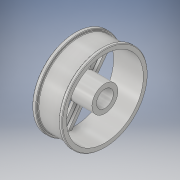
# Autodesk Inventor part: T9 Rim
Saved by Autodesk Inventor 2018 (Build 220112000, 112)
## iProperties
Created: 2018-02-18
Part Number: T9 Rim
Material: Phenolic Resin
Document SubType Name: Modeling
Designer: Blue Mist
Density: 1.38 g/cm^3
Appearance: Smooth - Light Orange
Author: Blue Mist
Autodesk Inventor part; units mm, degrees
ref_plane "YZ Plane" through (0, 0, 0) normal (1, 0, 0) x (0, 1, 0)
ref_plane "XZ Plane" through (0, 0, 0) normal (0, 1, 0) x (-1, 0, 0)
ref_plane "XY Plane" through (0, 0, 0) normal (0, 0, 1) x (1, 0, 0)
sketch "Sketch1" plane through (0, 0, 0) normal (0, 0, 1) x (1, 0, 0)
  line L0 (0, 0) -> (0, 17.653) construction
  line L1 (0, 17.907) -> (0, 21.209)
  line L2 (0.254, 21.463) -> (1.524, 21.463)
  line L3 (1.778, 21.209) -> (1.778, 18.923)
  line L4 (2.032, 18.669) -> (12.192, 18.669)
  line L5 (12.446, 18.923) -> (12.446, 21.209)
  line L6 (12.7, 21.463) -> (13.97, 21.463)
  line L7 (14.224, 21.209) -> (14.224, 17.907)
  line L8 (13.97, 17.653) -> (0.254, 17.653)
  arc A0 (13.97, 17.653) -> (14.224, 17.907) centre (13.97, 17.907) ccw
  arc A1 (14.224, 21.209) -> (13.97, 21.463) centre (13.97, 21.209) ccw
  arc A2 (12.7, 21.463) -> (12.446, 21.209) centre (12.7, 21.209) ccw
  arc A3 (12.192, 18.669) -> (12.446, 18.923) centre (12.192, 18.923) ccw
  arc A4 (1.778, 18.923) -> (2.032, 18.669) centre (2.032, 18.923) ccw
  arc A5 (1.778, 21.209) -> (1.524, 21.463) centre (1.524, 21.209) ccw
  arc A6 (0.254, 21.463) -> (0, 21.209) centre (0.254, 21.209) ccw
  arc A7 (0, 17.907) -> (0.254, 17.653) centre (0.254, 17.907) ccw
  line L9 (-2.9184, 0) -> (17.1424, 0) projected
  point P0 (0, 21.463)
  point P1 (1.778, 21.463)
  point P2 (1.778, 18.669)
  point P3 (12.446, 18.669)
  point P4 (12.446, 21.463)
  point P5 (14.224, 21.463)
  point P6 (14.224, 17.653)
  dimension "d0" = 17.653
  dimension "d1" = 3.81
  dimension "d2" = 1.778
  dimension "d3" = 2.794
  dimension "d4" = 10.668
  dimension "d5" = 2.794
  dimension "d6" = 1.778
  dimension "d7" = 3.81
  dimension "d8" = 0.254
  constraints: 19 point on line, 18 end point, 16 point on circle, 16 tangent, 8 centre point, 7 equal radius, 3 perpendicular, 1 parallel, 1 vertical
  measures "d0" distance of L0.start L0.end
  measures "d1" distance of L0.end point (0, 21.463)
  measures "d2" distance of point (0, 21.463) point (1.778, 21.463)
  measures "d3" distance of point (1.778, 21.463) point (1.778, 18.669)
  measures "d4" distance of point (1.778, 18.669) point (12.446, 18.669)
  measures "d5" distance of point (12.446, 18.669) point (12.446, 21.463)
  measures "d6" distance of point (12.446, 21.463) point (14.224, 21.463)
  measures "d7" distance of point (14.224, 21.463) point (14.224, 17.653)
  measures "d8" radius of A0
revolve "Revolution1" add sketch "Sketch1" angle 360 about axis through (-10, 0, 0) along (1, 0, 0)
sketch "Sketch2" plane through (0, 0, 0) normal (0, 0, 1) x (1, 0, 0)
  line L0 (0.254, -17.653) -> (0.254, 17.653) projected
  line L1 (0, -17.907) -> (0, 17.907) projected
  line L2 (0, -21.209) -> (0, 21.209) projected
  line L3 (13.97, -17.653) -> (13.97, 17.653) projected
  line L4 (0.254, -17.653) -> (0.254, 17.653) projected
  line L5 (13.97, 17.653) -> (0.254, 17.653) projected
  arc A0 (0.254, 21.463) -> (0, 21.209) centre (0.254, 21.209) ccw projected
  line L6 (0.254, 21.463) -> (1.524, 21.463) projected
  line L7 (0, -21.209) -> (0, 21.209) projected
  line L8 (0.254, -21.463) -> (0.254, 21.463) projected
  line L9 (1.524, -21.463) -> (1.524, 21.463) projected
  line L10 (1.778, -21.209) -> (1.778, 21.209) projected
  line L11 (14.224, -17.907) -> (14.224, 17.907) projected
  line L12 (1.524, -21.463) -> (1.524, 21.463) projected
  line L13 (14.224, -21.209) -> (14.224, 21.209) projected
  line L14 (0, 17.8534) -> (2.54, 5.969)
  line L15 (2.54, 5.969) -> (2.54, 3.8735)
  line L16 (2.54, 3.8735) -> (14.224, 3.8735)
  line L17 (14.224, 3.8735) -> (14.224, 5.969)
  line L18 (0, 17.8534) -> (1.27, 17.8534) construction
  line L19 (2.54, 5.969) -> (3.81, 5.969) construction
  line L20 (1.27, 17.653) -> (3.81, 5.969)
  line L21 (14.224, 5.969) -> (3.81, 5.969)
  line L22 (0, 17.8534) -> (1.27, 17.653)
  line L23 (-2.9079, 0) -> (17.0793, 0) projected
  point P0 (0, 0)
  dimension "d10" = 2.54
  dimension "d11" = 13.7795
  dimension "d12" = 2.54
  dimension "d13" = 11.684
  dimension "d14" = 1.27
  constraints: 18 end point, 4 point on line, 2 collinear, 2 perpendicular, 1 parallel
  measures "d10" distance from line of L1 L15.end
  measures "d11" distance from line of L5 L15.end
  measures "d12" distance from line of L1 L14.end
  measures "d13" distance from line of L5 L14.end
  measures "d14" distance of L14.end L19.end
revolve "Revolution2" add sketch "Sketch2" angle 360 about axis through (-10, 0, 0) along (1, 0, 0) contours L14 L22 L8 L0 | L0 L5 L20 L9 L14 | L8 L22 L5 | L9 L20 L10 L14 | L10 L20 L21 L3 L16 L15 L14 | L3 L21 L11 L16
sketch "Sketch3" plane through (0, 0, 0) normal (-1, 0, 0) x (0, 0, 1)
  circle A0 centre (0, 0) radius 17.8534 construction
  circle A1 centre (0, 0) radius 5.969 construction
  line L0 (5.969, 1.016) -> (5.8819, 1.016)
  circle A2 centre (0, 0) radius 5.969 projected
  line L1 (5.969, -1.016) -> (5.8819, -1.016)
  line L2 (5.969, -1.016) -> (17.6237, -1.016)
  circle A3 centre (0, 0) radius 17.653 projected
  line L3 (5.969, 1.016) -> (17.6237, 1.016)
  arc A4 (17.6237, -1.016) -> (17.6237, 1.016) centre (0, 0) ccw
  arc A5 (5.8819, -1.016) -> (5.8819, 1.016) centre (0, 0) ccw
  dimension "d16" = 1.016
  dimension "d17" = 1.016
  constraints: 8 end point, 8 point on circle, 2 centre point, 2 concentric, 2 horizontal, 2 parallel
  measures "d16" vertical distance of point (0, 0) L0.start
  measures "d17" vertical distance of point (0, 0) L1.start
extrude "Extrusion1" cut sketch "Sketch3" against normal blind 25.4 contours L3 A3 L2 L1 A2 L0 picked at (9.8507, 0.7907)
pattern_circular "Circular Pattern1" count 5 over 360 about axis through (-10, 0, 0) along (1, 0, 0) of "Extrusion1"
sketch "Sketch4" plane through (0, 0, 0) normal (-1, 0, 0) x (0, 0, 1)
  line L0 (-5.3557, 2.6353) -> (-14.8551, 9.537) projected
  line L1 (-14.8551, -9.537) -> (-5.3557, -2.6353) projected
  arc A0 (-14.8551, 9.537) -> (-14.8551, -9.537) centre (0, 0) ccw projected
  arc A1 (-5.3557, 2.6353) -> (-5.3557, -2.6353) centre (0, 0) ccw projected
  line L2 (-14.4076, 7.0142) -> (-7.1395, 1.7336)
  line L3 (-7.1395, 1.7336) -> (-5.9096, 0.84)
  arc A2 (-5.3557, 2.6353) -> (-5.3557, -2.6353) centre (0, 0) ccw projected
  line L4 (-14.4076, 7.0142) -> (-15.7438, 7.985)
  line L5 (-14.0745, -6.7722) -> (-7.4288, -1.9438)
  line L6 (-7.4288, -1.9438) -> (-5.9096, -0.84)
  line L7 (-14.0745, -6.7722) -> (-15.7438, -7.985)
  arc A3 (-5.9096, 0.84) -> (-5.9096, -0.84) centre (0, 0) ccw
  arc A4 (-15.7438, 7.985) -> (-15.7438, -7.985) centre (0, 0) ccw
  dimension "d23" = 1.778
  dimension "d24" = 1.778
  dimension "d25" = 1.778
  dimension "d26" = 1.778
  constraints: 12 end point, 7 point on circle, 3 point on line, 2 centre point
  measures "d23" distance from line of L0 L2.end
  measures "d24" distance from line of L0 L2.start
  measures "d25" distance from line of L1 L5.end
  measures "d26" distance from line of L1 L5.start
extrude "Extrusion2" cut sketch "Sketch4" against normal blind 25.4 contours A1 L6 L5 L7 A0 L4 L2 L3
pattern_circular "Circular Pattern2" count 5 over 360 about axis through (-10, 0, 0) along (1, 0, 0) of "Extrusion2"
sketch "Sketch5" plane through (14.224, 0, 0) normal (1, 0, 0) x (0, 0, -1)
  circle A0 centre (0, 0) radius 21.463 projected
extrude "Extrusion3" cut sketch "Sketch5" against normal blind 0.508
sketch "Sketch6" plane through (12.446, 0, 0) normal (-1, 0, 0) x (0, 0, 1)
  circle A0 centre (0, 0) radius 21.463 projected
extrude "Extrusion4" add sketch "Sketch6" along normal mid plane 0.508
sketch "Sketch7" plane through (12.7, 0, 0) normal (1, 0, 0) x (0, 0, -1)
  circle A0 centre (0, 0) radius 17.653 projected
  circle A1 centre (0, 0) radius 5.969 projected
  circle A2 centre (0, 0) radius 3.8735 projected
extrude "Extrusion5" cut sketch "Sketch7" against normal up to next
fillet "Fillet1" radius 0.254 3 edges at (12.192, 0, -21.463) (13.716, -21.463, 0) (12.192, -18.669, 0)
sketch "Sketch8" plane through (0, 0, 0) normal (-1, 0, 0) x (0, 0, 1)
  circle A0 centre (0, 0) radius 19.685
  circle A1 centre (0, 0) radius 21.463
  dimension "d39" = 39.37
  constraints: 2 centre point, 2 coincident
  measures "d39" diameter of A0
extrude "Extrusion6" cut sketch "Sketch8" against normal blind 508
fillet "Fillet2" radius 0.254 4 edges at (0, 0, -19.685) (1.778, 0, -19.685) (12.192, 0, -19.685) (13.716, 0, -19.685)
body "Solid1"
